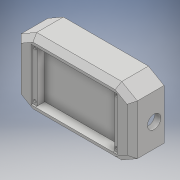
# Autodesk Inventor part: FSCase_Bottom_v6
Saved by Autodesk Inventor 2017 (Build 210142000, 142)
## iProperties
Created: 2020-03-11
Part Number: FSCase_Bottom_v6
Material: Generic
Document SubType Name: Modeling
Designer: Manny
Density: 1 g/cm^3
Appearance: Default
Author: Manny
Autodesk Inventor part; units mm, degrees
ref_plane "YZ Plane" through (0, 0, 0) normal (1, 0, 0) x (0, 1, 0)
ref_plane "XZ Plane" through (0, 0, 0) normal (0, 1, 0) x (-1, 0, 0)
sketch "Sketch1" plane through (0, 0, 0) normal (0, 1, 0) x (-1, 0, 0)
  line L0 (0, 0) -> (-95, 0)
  line L1 (-95, 0) -> (-95, -65)
  line L2 (-95, -65) -> (0, -65)
  line L3 (0, -65) -> (0, 0)
  line L4 (0, -65) -> (12.9904, -57.5)
  line L5 (12.9904, -57.5) -> (12.9904, -7.5)
  line L6 (12.9904, -7.5) -> (0, 0)
  line L7 (-95, -65) -> (-107.9904, -57.5)
  line L8 (-107.9904, -57.5) -> (-107.9904, -7.5)
  line L9 (-107.9904, -7.5) -> (-95, 0)
  dimension "d0" = 95
  dimension "d1" = 65
  dimension "d2" = 15
  dimension "d3" = 15
  dimension "d4" = 120
  dimension "d5" = 15
  dimension "d6" = 15
  dimension "d7" = 120
  constraints: 20 end point, 2 parallel, 2 vertical, 1 horizontal, 1 perpendicular
  measures "d0" distance of L0.start L0.end
  measures "d1" distance of L2.end L0.start
  measures "d2" distance of L2.end L4.end
  measures "d3" distance of L5.end L0.start
  measures "d4" angle of L5 L4
  measures "d5" distance of L1.end L7.end
  measures "d6" distance of L8.end L0.end
  measures "d7" angle of L8 L9
extrude "Extrusion1" add sketch "Sketch1" along normal blind 5
sketch "Sketch2" plane through (0, 5, 0) normal (0, 1, 0) x (1, 0, 0)
  line L0 (1.0001, 63.5) -> (94.0001, 63.5)
  line L1 (94.0001, 63.5) -> (94.0001, 1.5)
  line L2 (94.0001, 1.5) -> (1.0001, 1.5)
  line L3 (1.0001, 1.5) -> (1.0001, 63.5)
  line L4 (0, 0) -> (95, 0) projected
  line L5 (-12.9904, 57.5) -> (-12.9904, 7.5) projected
  dimension "d10" = 93
  dimension "d11" = 62
  dimension "d12" = 1.5
  dimension "d13" = 13.9905
  constraints: 8 end point, 2 parallel, 1 horizontal, 1 perpendicular
  measures "d10" distance of L0.start L0.end
  measures "d11" distance of L2.end L0.start
  measures "d12" distance between parallel lines of L4 L2
  measures "d13" distance between parallel lines of L5 L3
extrude "Extrusion2" add sketch "Sketch2" along normal blind 8
sketch "Sketch4" plane through (0, 5, 0) normal (0, 1, 0) x (1, 0, 0)
  line L0 (-12.9904, 57.5) -> (-12.9904, 7.5) projected
  line L1 (-12.9904, 57.5) -> (-12.9904, 7.5)
  line L2 (-12.9904, 7.5) -> (0, 0)
  line L3 (0, 0) -> (95, 0)
  line L4 (95, 0) -> (107.9904, 7.5) projected
  line L5 (95, 0) -> (107.9904, 7.5)
  line L6 (107.9904, 7.5) -> (107.9904, 57.5)
  line L7 (107.9904, 57.5) -> (95, 65) projected
  line L8 (107.9904, 57.5) -> (95, 65)
  line L9 (95, 65) -> (0, 65) projected
  line L10 (95, 65) -> (0, 65)
  line L11 (0, 65) -> (-12.9904, 57.5)
  line L12 (-19.9904, 61.5415) -> (-19.9904, 3.4585)
  line L13 (114.9904, 61.5415) -> (114.9904, 3.4585)
  line L14 (-1.8756, 72) -> (96.8756, 72)
  line L15 (-19.9904, 61.5415) -> (-1.8756, 72)
  line L16 (96.8756, 72) -> (114.9904, 61.5415)
  line L17 (114.9904, 3.4585) -> (96.8756, -7)
  line L18 (-19.9904, 3.4585) -> (-1.8756, -7)
  line L19 (-1.8756, -7) -> (96.8756, -7)
  line L20 (95, 0) -> (107.9904, 7.5) projected
  line L21 (107.9904, 7.5) -> (107.9904, 57.5) projected
  line L22 (0, 0) -> (95, 0) projected
  dimension "d22" = 7
  dimension "d23" = 7
  dimension "d24" = 7
  dimension "d25" = 7
  dimension "d26" = 7
  dimension "d27" = 7
  dimension "d28" = 7
  dimension "d29" = 7
  constraints: 32 end point, 12 parallel, 3 vertical, 2 collinear, 1 horizontal, 1 perpendicular
  measures "d22" distance between parallel lines of L0 L12
  measures "d23" distance between parallel lines of L11 L15
  measures "d24" distance between parallel lines of L10 L14
  measures "d25" distance between parallel lines of L7 L16
  measures "d26" distance between parallel lines of L6 L13
  measures "d27" distance between parallel lines of L4 L17
  measures "d28" distance between parallel lines of L3 L19
  measures "d29" distance between parallel lines of L2 L18
extrude "Extrusion4" add sketch "Sketch4" along normal blind 32 and the other way blind 5
sketch "Sketch5" plane through (0, 0, 0) normal (0, -1, 0) x (1, 0, 0)
  line L0 (2.4999, -63) -> (92.4999, -63)
  line L1 (92.4999, -63) -> (92.4999, -2)
  line L2 (92.4999, -2) -> (2.4999, -2)
  line L3 (2.4999, -2) -> (2.4999, -63)
  line L4 (0, 0) -> (95, 0) projected
  line L5 (-12.9904, -57.5) -> (-12.9904, -7.5) projected
  line L6 (96.8756, 7) -> (-1.8756, 7) projected
  line L7 (114.9904, -61.5415) -> (114.9904, -3.4585) projected
  line L8 (-1.8756, -72) -> (96.8756, -72) projected
  dimension "d34" = 61
  dimension "d35" = 90
  dimension "d44" = 22.4905
  dimension "d128" = 9
  constraints: 8 end point, 2 parallel, 1 horizontal, 1 perpendicular
  measures "d34" distance of L2.end L0.start
  measures "d35" distance of L1.end L2.end
  measures "d44" distance between parallel lines of L7 L1
  measures "d128" distance between parallel lines of L8 L0
extrude "Extrusion5" cut sketch "Sketch5" against normal blind 11
chamfer "Chamfer1" distance 6 angle 45 8 edges at (47.5, 0, -72) (105.933, 0, -66.7707) (114.9904, 0, -32.5) (105.933, 0, 1.7707) (47.5, 0, 7) (-10.933, 0, 1.7707) (-19.9904, 0, -32.5) (-10.933, 0, -66.7707)
sketch "Sketch6" plane through (0, 0, 0) normal (0, -1, 0) x (1, 0, 0)
  line L0 (2.4999, -2) -> (-2.5001, -2)
  line L1 (-2.5001, -2) -> (-2.5001, -63.0139)
  line L2 (-2.5001, -63.0139) -> (2.4999, -63.0139)
  line L3 (2.4999, -63.0139) -> (2.4999, -2)
  line L4 (2.4999, -2) -> (92.4999, -2) projected
  line L5 (92.4999, -2) -> (97.4999, -2)
  line L6 (97.4999, -2) -> (97.4999, -63.0139)
  line L7 (97.4999, -63.0139) -> (92.4999, -63.0139)
  line L8 (92.4999, -63.0139) -> (92.4999, -2)
  point P0 (0, 0)
  dimension "d45" = 5
  dimension "d46" = 5
  constraints: 16 end point, 4 parallel, 2 horizontal, 2 perpendicular
  measures "d45" distance of L1.end L2.end
  measures "d46" distance of L6.end L7.end
extrude "Extrusion6" cut sketch "Sketch6" against normal blind 2
sketch "Sketch7" plane through (0, 2, 0) normal (0, -1, 0) x (1, 0, 0)
  circle A0 centre (-0.0001, -6) radius 1.6
  circle A1 centre (94.9999, -6) radius 1.6
  circle A2 centre (-0.0001, -59.0139) radius 1.6
  circle A3 centre (94.9999, -59.0139) radius 1.6
  line L0 (94.0001, -63.5) -> (94.0001, -1.5) projected
  line L1 (2.4999, -2) -> (2.4999, -63) projected
  line L2 (97.4999, -2) -> (97.4999, -63.0139) projected
  line L3 (-2.5001, -2) -> (97.4999, -2) projected
  line L4 (-2.5001, -63.0139) -> (-2.5001, -2) projected
  line L5 (2.4999, -63.0139) -> (-2.5001, -63.0139) projected
  line L6 (92.4999, -63) -> (92.4999, -2) projected
  line L7 (97.4999, -63.0139) -> (92.4999, -63.0139) projected
  point P0 (0, 0)
  dimension "d49" = 3.2
  dimension "d50" = 2.5
  dimension "d51" = 2.5
  dimension "d52" = 4
  dimension "d53" = 0
  dimension "d54" = 2.5
  dimension "d55" = 4
  dimension "d56" = 2.5
  dimension "d57" = 4
  constraints: 4 centre point, 3 equal radius
  measures "d49" diameter of A0
  measures "d50" distance from line of L1 A0.centre
  measures "d51" distance from line of L2 A1.centre
  measures "d52" distance from line of L3 A0.centre
  measures "d53" vertical distance of A0.centre A1.centre
  measures "d54" distance from line of L4 A2.centre
  measures "d55" distance from line of L5 A2.centre
  measures "d56" distance from line of L6 A3.centre
  measures "d57" distance from line of L7 A3.centre
extrude "Extrusion7" cut sketch "Sketch7" against normal blind 1 contours A0 | A1 L0 | L0 A1 | L0 A3 | A3 L0 | A2
sketch "Sketch8" plane through (0, 13, 0) normal (0, 1, 0) x (1, 0, 0)
  line L0 (5.0001, 60.5) -> (90.0001, 60.5)
  line L1 (90.0001, 60.5) -> (90.0001, 4.5)
  line L2 (90.0001, 4.5) -> (5.0001, 4.5)
  line L3 (5.0001, 4.5) -> (5.0001, 60.5)
  line L4 (96.8756, 72) -> (-1.8756, 72) projected
  line L5 (-19.9904, 61.5415) -> (-19.9904, 3.4585) projected
  circle A0 centre (28.5001, 57) radius 2.5
  circle A1 centre (28.5001, 8) radius 2.5
  circle A2 centre (86.5001, 57) radius 2.5
  circle A3 centre (86.5001, 8) radius 2.5
  circle A4 centre (28.5001, 8) radius 1.6
  circle A5 centre (86.5001, 8) radius 1.6
  circle A6 centre (86.5001, 57) radius 1.6
  circle A7 centre (28.5001, 57) radius 1.6
  circle A8 centre (28.5001, 57) radius 2.5
  point P0 (0, 0)
  dimension "d60" = 85
  dimension "d61" = 56
  dimension "d62" = 11.5
  dimension "d63" = 24.9905
  dimension "d65" = 3.5
  dimension "d66" = 5
  dimension "d68" = 3.5
  dimension "d69" = 3.5
  dimension "d70" = 3.5
  dimension "d71" = 58
  dimension "d72" = 58
  dimension "d75" = 3.5
  dimension "d76" = 3.5
  dimension "d100" = 3.2
  dimension "d101" = 3.2
  dimension "d102" = 3.2
  dimension "d103" = 3.2
  constraints: 9 centre point, 8 end point, 5 coincident, 4 equal radius, 2 parallel, 1 horizontal, 1 perpendicular
  measures "d60" distance of L0.start L0.end
  measures "d61" distance of L2.end L0.start
  measures "d62" distance between parallel lines of L4 L0
  measures "d63" distance between parallel lines of L5 L3
  measures "d65" distance from line of L0 A0.centre
  measures "d66" diameter of A0
  measures "d68" distance from line of L2 A1.centre
  measures "d69" distance from line of L2 A3.centre
  measures "d70" distance from line of L0 A2.centre
  measures "d71" distance of A2.centre A0.centre
  measures "d72" distance of A3.centre A1.centre
  measures "d75" distance from line of L1 A2.centre
  measures "d76" distance from line of L1 A3.centre
  measures "d100" diameter of A7
  measures "d101" diameter of A6
  measures "d102" diameter of A4
  measures "d103" diameter of A5
extrude "Extrusion8" add sketch "Sketch8" along normal blind 5 contours A0 | A1 | A2 | A3 | A4 | A5 | A6 | A7
sketch "Sketch9" plane through (92.4999, 11, -63) normal (-1, 0, 0) x (0, 0, 1)
  circle A0 centre (49, -3) radius 1.5
  line L0 (61, 0) -> (0, 0) projected
  line L1 (61, -9) -> (61, 0) projected
  point P0 (63, -11)
  dimension "d77" = 3
  dimension "d78" = 3
  dimension "d79" = 12
  constraints: 1 centre point
  measures "d77" diameter of A0
  measures "d78" distance from line of L0 A0.centre
  measures "d79" distance from line of A0.centre L1
extrude "Extrusion9" cut sketch "Sketch9" against normal blind 5
sketch "Sketch10" plane through (0, 37, 0) normal (0, 1, 0) x (1, 0, 0)
  line L0 (-12.9904, 7.5) -> (-12.9904, 57.5) projected
  line L1 (-12.9904, 7.5) -> (-16.4904, 1.4378)
  line L2 (-1.8756, -7) -> (-19.9904, 3.4585) projected
  line L3 (0, 0) -> (95, 0) projected
  line L4 (0, 0) -> (-3.486, -6.038)
  line L5 (-12.9904, 57.5) -> (0, 65) projected
  line L6 (-12.9904, 57.5) -> (-16.4904, 63.5622)
  line L7 (-1.8756, 72) -> (-19.9904, 61.5415) projected
  line L8 (0, 65) -> (-3.5, 71.0622)
  line L9 (0, 65) -> (95, 65) projected
  line L10 (95, 65) -> (98.5, 71.0622)
  line L11 (114.9904, 61.5415) -> (96.8756, 72) projected
  line L12 (107.9904, 57.5) -> (95, 65) projected
  line L13 (107.9904, 57.5) -> (111.4904, 63.5622)
  line L14 (95, 0) -> (107.9904, 7.5) projected
  line L15 (107.9904, 7.5) -> (111.4904, 1.4378)
  line L16 (95, 0) -> (98.5, -6.0622)
  line L17 (96.8756, -7) -> (114.9904, 3.4585) projected
  circle A0 centre (103.2452, 0.7189) radius 1.85
  circle A1 centre (103.2452, 64.2811) radius 1.6
  circle A2 centre (-8.2452, 64.2811) radius 1.65
  circle A3 centre (-8.2452, 0.7189) radius 1.75
  circle A4 centre (46.5, -3.5) radius 1.8
  circle A5 centre (46.5, 68.5) radius 1.7
  line L18 (0, 0) -> (-12.9904, 7.5) projected
  line L19 (-12.9904, 7.5) -> (0, 0) projected
  line L20 (0, 0) -> (0, -7)
  line L21 (-1.8756, -7) -> (96.8756, -7) projected
  line L22 (0, 65) -> (0, 72)
  dimension "d82" = 3.2
  dimension "d83" = 7.5
  dimension "d84" = 90
  dimension "d85" = 3.5
  dimension "d86" = 90
  dimension "d87" = 7.5
  dimension "d88" = 3.5
  dimension "d89" = 7.5
  dimension "d90" = 3.5
  dimension "d91" = 7.5
  dimension "d92" = 3.5
  dimension "d93" = 46.5
  dimension "d95" = 46.5
  dimension "d96" = 3.5
  dimension "d97" = 3.5
  dimension "d129" = 3.4
  dimension "d130" = 3.3
  dimension "d131" = 3.5
  dimension "d132" = 3.7
  dimension "d133" = 3.6
  constraints: 20 end point, 7 point on line, 6 centre point, 5 parallel, 1 perpendicular, 1 vertical
  measures "d82" diameter of A1
  measures "d83" distance from line of L13 A1.centre
  measures "d84" angle of L11 L13
  measures "d85" distance from line of L12 A1.centre
  measures "d86" angle of L7 L6
  measures "d87" distance from line of A2.centre L6
  measures "d88" distance from line of L5 A2.centre
  measures "d89" distance from line of L1 A3.centre
  measures "d90" distance from line of L18 A3.centre
  measures "d91" distance from line of L15 A0.centre
  measures "d92" distance from line of L14 A0.centre
  measures "d93" distance from line of L20 A4.centre
  measures "d95" distance from line of L22 A5.centre
  measures "d96" distance from line of L9 A5.centre
  measures "d97" distance from line of L3 A4.centre
  measures "d129" diameter of A5
  measures "d130" diameter of A2
  measures "d131" diameter of A3
  measures "d132" diameter of A0
  measures "d133" diameter of A4
extrude "Extrusion10" cut sketch "Sketch10" against normal blind 3 contours A0 | A1 | A2 | A3 | A4 | A5
ref_plane "Work Plane2" through (0, 18, 0) normal (0, 1, 0) x (1, 0, 0)
sketch "Sketch14" plane through (0, 18, 0) normal (0, 1, 0) x (1, 0, 0)
  circle A0 centre (28.5001, 8) radius 1.6
  circle A1 centre (28.5001, 8) radius 2.5 projected
  line L0 (28.5001, 8) -> (86.5001, 8)
  line L1 (86.5001, 8) -> (86.5001, 64)
  line L2 (86.5001, 64) -> (28.5001, 64)
  line L3 (28.5001, 64) -> (28.5001, 8)
  point P0 (0, 0)
  dimension "d108" = 3.2
  dimension "d109" = 0
  dimension "d110" = 0
  dimension "d117" = 56
  dimension "d118" = 58
  constraints: 8 end point, 2 parallel, 1 centre point, 1 horizontal, 1 perpendicular
  measures "d108" diameter of A0
  measures "d109" distance of L0.start A0.centre
  measures "d110" distance of L0.start A0.centre
  measures "d117" distance of L0.end L1.end
  measures "d118" distance of L0.start L0.end
extrude "Extrusion11" cut sketch "Sketch14" against normal blind 2.5 contours L0 L3 A0 | A0 L3 L0
sketch "Sketch15" plane through (86.5001, 18, -8) normal (0, 1, 0) x (1, 0, 0)
  circle A0 centre (0, 0) radius 1.6
  circle A1 centre (0, 49) radius 1.6
  circle A2 centre (0, 49) radius 2.5
  circle A3 centre (-58, 0) radius 1.6 projected
  line L0 (-58, 0) -> (0, 0)
  line L1 (0, 0) -> (0, 49)
  line L2 (0, 49) -> (-58, 49)
  line L3 (-58, 49) -> (-58, 0)
  circle A4 centre (-58, 49) radius 1.6
  point P0 (-86.5001, -8)
  dimension "d113" = 3.2
  dimension "d114" = 3.2
  dimension "d115" = 5
  dimension "d116" = 0
  dimension "d119" = 49
  dimension "d120" = 58
  dimension "d121" = 3.2
  constraints: 8 end point, 4 centre point, 2 parallel, 1 coincident, 1 horizontal, 1 perpendicular
  measures "d113" diameter of A0
  measures "d114" diameter of A1
  measures "d115" diameter of A2
  measures "d116" distance of L1.end A1.centre
  measures "d119" distance of L0.end L1.end
  measures "d120" distance of L0.start L0.end
  measures "d121" diameter of A4
extrude "Extrusion12" cut sketch "Sketch15" against normal blind 2.5 contours A0 L0 L1 | L1 L0 A0 | L1 L2 A1 | A1 L2 L1 | A4 L3 L2 | L2 L3 A4
sketch "Sketch16" plane through (107.9904, 5, -57.5) normal (-1, 0, 0) x (0, 0, 1)
  circle A0 centre (23.3152, 20.5) radius 7.8
  line L0 (0, 32) -> (50, 32) projected
  line L1 (0, 32) -> (50, 32)
  line L2 (57.5, 0) -> (50, 0) projected
  line L3 (50, 32) -> (50, 0)
  line L4 (50, 0) -> (0, 0)
  line L5 (0, 0) -> (0, 32) projected
  line L6 (0, 0) -> (0, 32)
  line L7 (-52.9421, -1.2141) -> (6.8536, -5)
  line L8 (6.8536, -5) -> (-57.6878, -5)
  line L9 (-57.6878, -5) -> (10.0174, -1.2141)
  point P0 (57.5, -5)
  dimension "d124" = 15.6
  dimension "d125" = 11.5
  constraints: 14 end point, 2 collinear, 2 perpendicular, 1 centre point, 1 horizontal
  measures "d124" diameter of A0
  measures "d125" distance from line of L0 A0.centre
extrude "Extrusion13" cut sketch "Sketch16" against normal blind 10 contours A0
body "Solid1"
